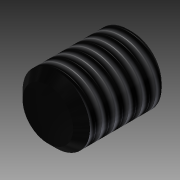
# Autodesk Inventor part: screw_M2_2
Saved by Autodesk Inventor 2013 (Build 170138000, 138)
## iProperties
Created: 2015-02-20
Part Number: screw_M2_2
Material: 一般
Document SubType Name: Modeling
Designer: Noa Izumi
Density: 1 g/cm^3
Author: Noa Izumi
Autodesk Inventor part; units mm, degrees
ref_plane "YZ Plane" through (0, 0, 0) normal (1, 0, 0) x (0, 1, 0)
ref_plane "XZ Plane" through (0, 0, 0) normal (0, 1, 0) x (-1, 0, 0)
ref_plane "XY Plane" through (0, 0, 0) normal (0, 0, 1) x (1, 0, 0)
sketch "草圖1" plane through (0, 0, 0) normal (0, 1, 0) x (-1, 0, 0)
  circle A0 centre (0, 0) radius 1
  dimension "d0" = 2
  constraints: 1 centre point, 1 coincident
  measures "d0" diameter of A0
extrude "擠出1" add sketch "草圖1" along normal blind 2.5
thread "螺紋1" size "M2x0.4" class "6g" standard "ANSI Metric M Profile" full length
chamfer "倒角1" distance 0.25 angle 45 1 edges at (1, 0, 0)
sketch "草圖2" plane through (0, 2.5, 0) normal (0, 1, 0) x (1, 0, 0)
  circle A0 centre (0, 0) radius 1 projected
  line L0 (0.3464, 0.6) -> (0.6928, 0)
  line L1 (0.6928, 0) -> (0.3464, -0.6)
  line L2 (0.3464, -0.6) -> (-0.3464, -0.6)
  line L3 (-0.3464, -0.6) -> (-0.6928, 0)
  line L4 (-0.6928, 0) -> (-0.3464, 0.6)
  line L5 (-0.3464, 0.6) -> (0.3464, 0.6)
  dimension "d9" = 1.2
  constraints: 12 end point, 1 coincident, 13 other
  measures "d9" distance between parallel lines of L2 L5
extrude "擠出2" cut sketch "草圖2" against normal blind 2 contours L0 L1 L2 L3 L4 L5
chamfer "倒角2" distance 0.125 angle 45 7 edges at (1, 2.5, 0) (0.5196, 2.5, -0.3) (0.5196, 2.5, 0.3) (0, 2.5, 0.6) (-0.5196, 2.5, 0.3) (-0.5196, 2.5, -0.3) (0, 2.5, -0.6)
